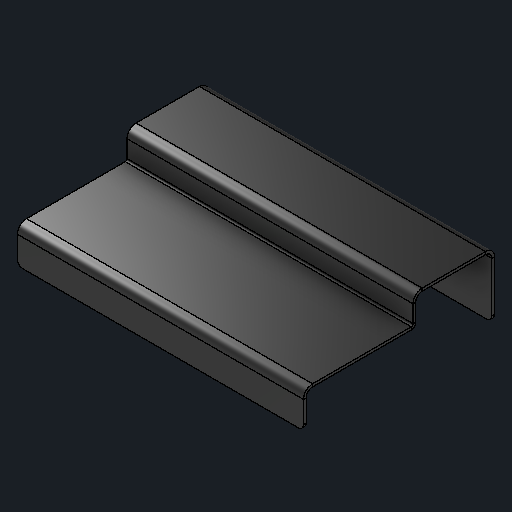
# Autodesk Inventor part: Top Shell
Saved by Autodesk Inventor 2026.2 (Build 302298000, 298)
## iProperties
Created: 2026-06-19
Part Number: Top Shell
Material: Steel, Carbon
Document SubType Name: Sheet Metal
Designer: JoshuaEah
Density: 7.85 g/cm^3
Sheet Metal Rule: Default_mm
Appearance: Glossy - Black
Author: JoshuaEah
Autodesk Inventor part; units mm, degrees
ref_plane "YZ Plane" through (0, 0, 0) normal (1, 0, 0) x (0, 1, 0)
ref_plane "XZ Plane" through (0, 0, 0) normal (0, 1, 0) x (-1, 0, 0)
ref_plane "XY Plane" through (0, 0, 0) normal (0, 0, 1) x (1, 0, 0)
sketch "Sketch1" plane through (0, 0, 0) normal (0, 1, 0) x (-1, 0, 0)
  line L0 (0, 0) -> (-158, 0)
  line L1 (-158, 0) -> (-158, -62)
  line L2 (-158, -62) -> (0, -62)
  line L3 (0, -62) -> (0, 0)
  dimension "d0" = 62
  dimension "d1" = 158
  measures "d0" distance of L0.end L1.end
  measures "d1" distance of L1.end L2.end
extrude "Plate1" add sketch "Sketch1" along normal blind 1.5
sketch "Sketch2" plane through (0, 0, -60.5) normal (0, 0, -1) x (-1, 0, 0)
  line L0 (-158, 0) -> (0, 0)
  line L1 (0, 0) -> (0, 17)
  line L2 (0, 17) -> (-158, 17)
  line L3 (-158, 17) -> (-158, 0)
  constraints: 6 end point, 1 horizontal, 1 perpendicular, 1 vertical
edge flange "Flange1" height 17 angle 90 thickness 1.5 bend radius 1 thickness toward (0, 0, -1) relief straight relief width 1.5 relief depth 0.75 edges at (79, 1.5, -62) wall of the first edge with corners at (158, 0, -60.5) (0, 0, -60.5) (0, 17, -60.5) (158, 17, -60.5)
bend "Bend1"
corner "Corner1"
sketch "Sketch3" plane through (0, 1.5, -1.5) normal (0, 0, 1) x (1, 0, 0)
  line L0 (158, 0) -> (0, 0)
  line L1 (0, 0) -> (0, -20)
  line L2 (0, -20) -> (158, -20)
  line L3 (158, -20) -> (158, 0)
  constraints: 6 end point, 1 horizontal, 1 perpendicular, 1 vertical
edge flange "Flange2" height 20 angle 90 thickness 1.5 bend radius 3.5 thickness toward (0, 0, 1) relief straight relief width 1.5 relief depth 0.75 edges at (79, 0, 0) wall of the first edge with corners at (158, 1.5, -1.5) (0, 1.5, -1.5) (0, -18.5, -1.5) (158, -18.5, -1.5)
bend "Bend2"
corner "Corner2"
sketch "Sketch4" plane through (158, 15.5, -60.5) normal (0, 1, 0) x (-1, 0, 0)
  line L0 (158, 0) -> (0, 0)
  line L1 (0, 0) -> (0, -45)
  line L2 (0, -45) -> (158, -45)
  line L3 (158, -45) -> (158, 0)
  constraints: 6 end point, 1 horizontal, 1 perpendicular, 1 vertical
edge flange "Flange3" height 45 angle 90 thickness 1.5 bend radius 3.5 thickness toward (0, 1, 0) relief straight relief width 1.5 relief depth 0.75 edges at (79, 17, -62) wall of the first edge with corners at (0, 15.5, -60.5) (158, 15.5, -60.5) (158, 15.5, -105.5) (0, 15.5, -105.5)
bend "Bend3"
corner "Corner3"
sketch "Sketch5" plane through (158, 17, -104) normal (0, 0, -1) x (-1, 0, 0)
  line L0 (158, 0) -> (0, 0)
  line L1 (0, 0) -> (0, -35.5)
  line L2 (0, -35.5) -> (158, -35.5)
  line L3 (158, -35.5) -> (158, 0)
  constraints: 6 end point, 1 horizontal, 1 perpendicular, 1 vertical
edge flange "Flange4" height 35.5 angle 90 thickness 1.5 bend radius 3.5 thickness toward (0, 0, -1) relief straight relief width 1.5 relief depth 0.75 edges at (79, 15.5, -105.5) wall of the first edge with corners at (0, 17, -104) (158, 17, -104) (158, -18.5, -104) (0, -18.5, -104)
bend "Bend4"
corner "Corner4"
fillet "Fillet1" radius 3 4 edges at (158, -18.5, -0.75) (0, -18.5, -0.75) (0, -18.5, -104.75) (158, -18.5, -104.75)
equation "\"d2\" = Thickness"
equation "\"d3\" = BendReliefWidth"
equation "\"d4\" = BendReliefDepth"
equation "\"d5\" = MinimumRemnant"
equation "\"d6\" = TransitionRadius"
equation "\"d10\" = CornerReliefSize"
equation "\"d11\" = GapSize"
equation "\"d12\" = JacobiRadiusSize"
equation "\"d13\" = BendReliefWidth"
equation "\"d14\" = BendReliefDepth"
equation "\"d15\" = MinimumRemnant"
equation "\"d16\" = TransitionRadius"
equation "\"d20\" = CornerReliefSize"
equation "\"d21\" = GapSize"
equation "\"d22\" = JacobiRadiusSize"
equation "\"d23\" = BendReliefWidth"
equation "\"d24\" = BendReliefDepth"
equation "\"d25\" = MinimumRemnant"
equation "\"d26\" = TransitionRadius"
equation "\"d30\" = CornerReliefSize"
equation "\"d31\" = GapSize"
equation "\"d32\" = JacobiRadiusSize"
equation "\"d33\" = BendReliefWidth"
equation "\"d34\" = BendReliefDepth"
equation "\"d35\" = MinimumRemnant"
equation "\"d36\" = TransitionRadius"
equation "\"d40\" = CornerReliefSize"
equation "\"d41\" = GapSize"
equation "\"d42\" = JacobiRadiusSize"
equation "\"BendRadius\" = Thickness"
equation "\"BendReliefWidth\" = Thickness"
equation "\"BendReliefDepth\" = 0.5 * Thickness"
equation "\"CornerReliefSize\" = 4 * Thickness"
equation "\"MinimumRemnant\" = 2 * Thickness"
equation "\"TransitionRadius\" = BendRadius"
equation "\"JacobiRadiusSize\" = BendRadius"
equation "\"GapSize\" = Thickness"
equation "\"Thickness\" = 1.5"
body "Solid1"
